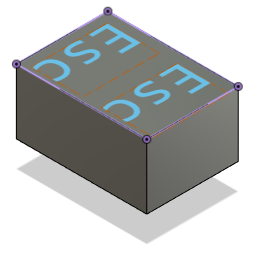
Key Cap v12 (Autodesk Fusion 360 design; units mm, degrees)
Autodesk Fusion 360 part; units mm, degrees
sketch "Sketch1" plane through (0, 0, 0) normal (0, 1, 0) x (1, 0, 0)
  line L0 (12.4312, -14.3607) -> (13.4312, -14.3607)
  line L1 (13.4312, -14.3607) -> (13.4312, -17.3607)
  line L2 (13.4312, -17.3607) -> (12.4312, -17.3607)
  line L3 (12.4312, -17.3607) -> (12.4312, -14.3607)
  line L4 (12.9312, -14.3607) -> (12.9312, -17.3607) construction
  line L5 (12.4312, -15.8607) -> (13.4312, -15.8607) construction
  line L6 (13.4312, -15.8607) -> (18.2312, -15.8607) construction
  line L7 (18.2312, -14.3607) -> (18.2312, -17.3607) construction
  line L8 (17.7312, -14.3607) -> (18.7312, -14.3607)
  line L9 (18.7312, -14.3607) -> (18.7312, -17.3607)
  line L10 (18.7312, -17.3607) -> (17.7312, -17.3607)
  line L11 (17.7312, -17.3607) -> (17.7312, -14.3607)
  line L12 (9.8312, -10.8607) -> (21.8312, -10.8607)
  line L13 (21.8312, -10.8607) -> (21.8312, -22.2607)
  line L14 (21.8312, -22.2607) -> (9.8312, -22.2607)
  line L15 (9.8312, -22.2607) -> (9.8312, -10.8607)
  line L16 (15.8312, -10.8607) -> (15.8312, -22.2607) construction
  line L17 (21.8312, -16.5607) -> (9.8312, -16.5607) construction
  line L18 (10.0312, -12.2607) -> (21.6312, -12.2607)
  line L19 (21.6312, -12.2607) -> (21.6312, -20.8607)
  line L20 (21.6312, -20.8607) -> (10.0312, -20.8607)
  line L21 (10.0312, -20.8607) -> (10.0312, -12.2607)
  line L22 (10.8012, -13.0307) -> (20.8612, -13.0307)
  line L23 (20.8612, -13.0307) -> (20.8612, -20.0907)
  line L24 (20.8612, -20.0907) -> (10.8012, -20.0907)
  line L25 (10.8012, -20.0907) -> (10.8012, -13.0307)
  point P0 (15.8312, -15.8607)
  point P1 (21.6312, -16.5607)
  point P2 (15.8312, -12.2607)
  dimension "d3" = 1
  dimension "d4" = 3
  dimension "d6" = 1
  dimension "d7" = 3
  dimension "d8" = 5.3
  dimension "d9" = 12
  dimension "d10" = 11.4
  dimension "d11" = 5
  dimension "d14" = 11.6
  dimension "d15" = 8.6
  dimension "d17" = 0.77
  dimension "d18" = 0.77
  dimension "d19" = 0.77
  dimension "d20" = 0.77
  constraint horizontal L0
  constraint vertical L1
  constraint horizontal L2
  constraint vertical L3
  constraint midpoint L0 L4.start
  constraint midpoint L2 L4.end
  constraint midpoint L3 L5.start
  constraint midpoint L1 L5.end
  constraint perpendicular L1 L6
  constraint perpendicular L6 L7
  constraint horizontal L8
  constraint vertical L9
  constraint horizontal L10
  constraint vertical L11
  constraint midpoint L7.start L8
  constraint midpoint L7.end L10
  constraint midpoint L6.end L7
  constraint horizontal L12
  constraint vertical L13
  constraint horizontal L14
  constraint vertical L15
  constraint midpoint L12 L16.start
  constraint midpoint L14 L16.end
  constraint midpoint L6 P0
  constraint coincident L16 P0
  constraint midpoint L13 L17.start
  constraint midpoint L15 L17.end
  constraint horizontal L18
  constraint vertical L19
  constraint horizontal L20
  constraint vertical L21
  constraint midpoint L19 P1
  constraint coincident L17 P1
  constraint midpoint L18 P2
  constraint coincident L16 P2
  constraint horizontal L22
  constraint vertical L23
  constraint horizontal L24
  constraint vertical L25
  measures "d3" distance of L0.start L0.end
  measures "d4" distance of L0.start L2.end
  measures "d6" distance of L8.start L8.end
  measures "d7" distance of L8.start L10.end
  measures "d8" distance of L4 L7
  measures "d9" distance of L12.start L12.end
  measures "d10" distance of L12.start L14.end
  measures "d11" distance of L6 L12
  measures "d14" distance of L18.start L18.end
  measures "d15" distance of L18.start L20.end
  measures "d17" distance of L18 L22
  measures "d18" distance of L19 L23
  measures "d19" distance of L20 L24
  measures "d20" distance of L21 L25
extrude "Extrude1" add sketch "Sketch1" along normal blind 2 contours L0 L1 L2 L3 | L8 L9 L10 L11 makes body 1 at (13.4312, 0.6667, 15.3607) makes body 2 at (18.7312, 0.6667, 15.3607)
extrude "Extrude2" add sketch "Sketch1" along normal blind 5 from surface at 2 contours L0 L1 L2 L3 | L8 L9 L10 L11 | L22 L23 L24 L25 bodies 1 2
fillet "Fillet1" [suppressed]
sketch "Sketch2" plane through (0, 7, 0) normal (0, 1, 0) x (-1, 0, 0)
  line L0 (-16.9627, 13.8658) -> (-16.9627, 19.7076) construction
  line L1 (-16.9627, 19.7076) -> (-20.9627, 19.7076) construction
  line L2 (-20.9627, 19.7076) -> (-20.9627, 13.8658) construction
  line L3 (-20.9627, 13.8658) -> (-16.9627, 13.8658) construction
  line L4 (-11.5741, 13.8658) -> (-11.5741, 19.7076) construction
  line L5 (-11.5741, 19.7076) -> (-15.5741, 19.7076) construction
  line L6 (-15.5741, 19.7076) -> (-15.5741, 13.8658) construction
  line L7 (-15.5741, 13.8658) -> (-11.5741, 13.8658) construction
  line L8 (-10.8012, 13.0307) -> (-10.8012, 20.0907)
  line L9 (-10.8012, 20.0907) -> (-20.8612, 20.0907)
  line L10 (-20.8612, 20.0907) -> (-20.8612, 13.0307)
  line L11 (-20.8612, 13.0307) -> (-10.8012, 13.0307)
  constraint perpendicular L0 L1
  constraint parallel L0 L2
  constraint parallel L1 L3
  constraint perpendicular L4 L5
  constraint parallel L4 L6
  constraint parallel L5 L7
extrude "Extrude3" [suppressed]
extrude "Extrude4" [suppressed]
equation "PostW = 1 mm"
equation "PostH = 3 mm"
equation "d3 = PostW"
equation "d4 = PostH"
equation "d6 = PostW"
equation "d7 = PostH"
equation "HoleW = 8.6 mm"
equation "HoleH = 11.6 mm"
equation "d14 = HoleH"
equation "d15 = HoleW"
equation "HoleTol = 0.77 mm"
equation "d17 = HoleTol"
equation "d18 = HoleTol"
equation "d19 = HoleTol"
equation "d20 = HoleTol"
equation "CapD = 5 mm"
equation "PostD = 2 mm"
equation "d23 = PostD"
equation "d26 = CapD"
named bodies: "Key Cap"
